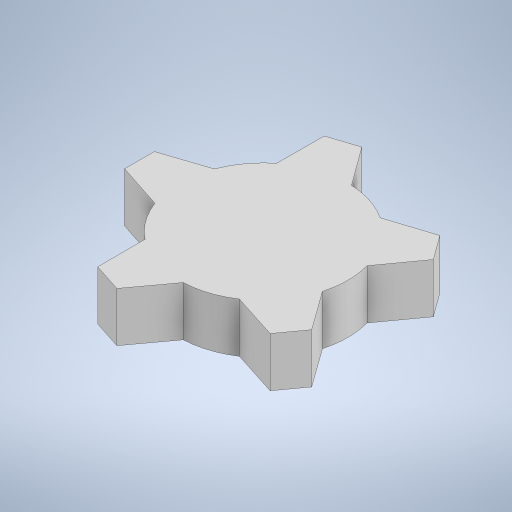
# Autodesk Inventor part: AP-1-01-spur5tooth
Saved by Autodesk Inventor 2023 (Build 270158000, 158)
## iProperties
Created: 2023-06-27
Part Number: AP-1-01-spur5tooth
Material: Generic
Document SubType Name: Modeling
Designer: t205b
Density: 1 g/cm^3
Appearance: Default
Author: t205b
Autodesk Inventor part; units mm, degrees
ref_plane "YZ Plane" through (0, 0, 0) normal (1, 0, 0) x (0, 1, 0)
ref_plane "XZ Plane" through (0, 0, 0) normal (0, 1, 0) x (-1, 0, 0)
ref_plane "XY Plane" through (0, 0, 0) normal (0, 0, 1) x (1, 0, 0)
sketch "Sketch1" plane through (0, 0, 0) normal (0, 1, 0) x (-1, 0, 0)
  circle A0 centre (0, 0) radius 8.5
  line L0 (7.953, 3) -> (12.5, 1.5)
  line L1 (12.5, 1.5) -> (12.5, -1.5)
  line L2 (12.5, -1.5) -> (7.953, -3)
  line L3 (5.2893, 11.4247) -> (5.3108, 6.6367)
  line L4 (-0.3956, 8.4908) -> (2.4361, 12.3517)
  line L5 (2.4361, 12.3517) -> (5.2893, 11.4247)
  line L6 (-9.231, 8.5608) -> (-4.6707, 7.1017)
  line L7 (-8.1975, 2.2476) -> (-10.9944, 6.1338)
  line L8 (-10.9944, 6.1338) -> (-9.231, 8.5608)
  line L9 (-10.9944, -6.1338) -> (-8.1975, -2.2476)
  line L10 (-4.6707, -7.1017) -> (-9.231, -8.5608)
  line L11 (-9.231, -8.5608) -> (-10.9944, -6.1338)
  line L12 (2.4361, -12.3517) -> (-0.3956, -8.4908)
  line L13 (5.3108, -6.6367) -> (5.2893, -11.4247)
  line L14 (5.2893, -11.4247) -> (2.4361, -12.3517)
  point P0 (-0.3956, -8.4908)
  dimension "d0" = 17
  dimension "d1" = 3
  dimension "d2" = 4
  dimension "d3" = 6
  dimension "d4" = 108.257
  dimension "d5" = 108.257
  dimension "d8" = 360
  constraints: 30 end point, 2 point on circle, 1 centre point, 1 coincident, 1 equal length, 1 vertical, 36 other
  measures "d0" diameter of A0
  measures "d1" distance of L0.end L1.end
  measures "d2" distance edge to line of A0 L1
  measures "d3" distance of L0.start L2.end
  measures "d4" angle of L2 L1
  measures "d5" angle of L0 L1
extrude "Extrusion1" add sketch "Sketch1" along normal blind 5
equation "\"d4\" = d5"
body "Solid1"
